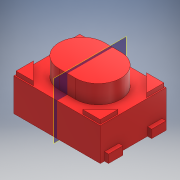
# Autodesk Inventor part: SKRPACE010
Saved by Autodesk Inventor 2018 (Build 220112000, 112)
## iProperties
Part Number: SKRPACE010
Material: 一般
Document SubType Name: Modeling
Designer: sktom
Density: 1 g/cm^3
Appearance: 淡い赤
Author: sktom
Autodesk Inventor part; units mm, degrees
ref_plane "YZ Plane" through (0, 0, 0) normal (1, 0, 0) x (0, 1, 0)
ref_plane "XZ Plane" through (0, 0, 0) normal (0, 1, 0) x (-1, 0, 0)
ref_plane "XY Plane" through (0, 0, 0) normal (0, 0, 1) x (1, 0, 0)
sketch "スケッチ1" plane through (0, 0, 0) normal (0, 0, 1) x (1, 0, 0)
  line L0 (-2.1, -1.6) -> (2.1, -1.6)
  line L1 (2.1, -1.6) -> (2.1, 1.6)
  line L2 (2.1, 1.6) -> (-2.1, 1.6)
  line L3 (-2.1, 1.6) -> (-2.1, -1.6)
  line L4 (-2.1, -1.6) -> (2.1, 1.6) construction
  line L5 (2.1, -1.6) -> (-2.1, 1.6) construction
  point P0 (0, 0)
  point P1 (0, 0)
  point P2 (0, 0)
  dimension "d0" = 4.2
  dimension "d1" = 3.2
  constraints: 12 end point, 3 midpoint, 2 parallel, 1 coincident, 1 horizontal, 1 perpendicular
  measures "d0" distance of L1.end L2.end
  measures "d1" distance of L0.end L1.end
extrude "押し出し1" add sketch "スケッチ1" along normal blind 1.6
sketch "スケッチ2" plane through (0, 0, 1.6) normal (0, 0, 1) x (1, 0, 0)
  line L0 (-0.4, 0) -> (0.4, 0) construction
  line L1 (-0.4, -1.1) -> (0.4, -1.1)
  line L2 (0.4, 1.1) -> (-0.4, 1.1)
  arc A0 (-0.4, 1.1) -> (-0.4, -1.1) centre (-0.4, 0) ccw
  arc A1 (0.4, -1.1) -> (0.4, 1.1) centre (0.4, 0) ccw
  point P0 (0, 0)
  point P1 (0, 0)
  dimension "d4" = 2.2
  dimension "d5" = 3
  constraints: 8 end point, 4 point on circle, 4 tangent, 2 centre point, 1 coincident, 1 horizontal, 1 midpoint, 1 parallel
  measures "d4" distance between parallel lines of L1 L2
extrude "押し出し2" add sketch "スケッチ2" along normal blind 0.9
sketch "スケッチ3" plane through (0, 0, 1.6) normal (0, 0, 1) x (1, 0, 0)
  line L0 (-2.05, 1.55) -> (-2.05, 0.7)
  line L1 (-2.05, 0.7) -> (-1.2, 1.55)
  line L2 (-1.2, 1.55) -> (-2.05, 1.55)
  line L3 (2.1, 1.6) -> (-2.1, 1.6) projected
  line L4 (-2.1, 1.6) -> (-2.1, -1.6) projected
  point P0 (0, 0)
  dimension "d8" = 0.05
  dimension "d9" = 0.05
  dimension "d10" = 0.7
  constraints: 6 end point, 1 horizontal, 1 perpendicular, 1 vertical
  measures "d8" distance between parallel lines of L3 L2
  measures "d9" distance between parallel lines of L4 L0
  measures "d10" vertical distance of point (0, 0) L0.end
extrude "押し出し3" add sketch "スケッチ3" along normal blind 0.2
mirror "ミラー1" about plane through (0, 0, 0) normal (1, 0, 0) of "押し出し3"
mirror "ミラー2" about plane through (0, 0, 0) normal (0, 1, 0) of "押し出し3", "ミラー1"
sketch "スケッチ4" plane through (0, 0, 0) normal (0, 0, -1) x (-1, 0, 0)
  line L0 (2.3, -1.4) -> (1.2, -1.4)
  line L1 (1.2, -1.4) -> (1.2, -0.7)
  line L2 (1.2, -0.7) -> (2.3, -0.7)
  line L3 (2.3, -0.7) -> (2.3, -1.4)
  line L4 (0, 2.24) -> (0, -2.24) projected
  line L5 (2.1, -1.6) -> (-2.1, -1.6) projected
  line L6 (2.1, 1.6) -> (2.1, -1.6) projected
  point P0 (0, 0)
  dimension "d13" = 2.3
  dimension "d14" = 0.7
  dimension "d15" = 0.2
  dimension "d16" = 0.9
  constraints: 8 end point, 2 parallel, 1 horizontal, 1 perpendicular
  measures "d13" distance between parallel lines of L4 L3
  measures "d14" distance from line of point (0, 0) L2
  measures "d15" distance between parallel lines of L0 L5
  measures "d16" distance between parallel lines of L6 L1
extrude "押し出し4" add sketch "スケッチ4" along normal blind 0.001 and the other way blind 0.4
mirror "ミラー3" about plane through (0, 0, 0) normal (-1, 0, 0) of "押し出し4"
mirror "ミラー4" about plane through (0, 0, 0) normal (0, 1, 0) of "押し出し4", "ミラー3"
ref_plane "作業平面1" through (0, 0, 0) normal (1, 0, 0) x (0, 1, 0)
ref_plane "作業平面2" through (0, 0, 0) normal (-1, 0, 0) x (0, -1, 0)
ref_plane "作業平面3" through (0, 0, 0) normal (-1, 0, 0) x (0, -1, 0)
